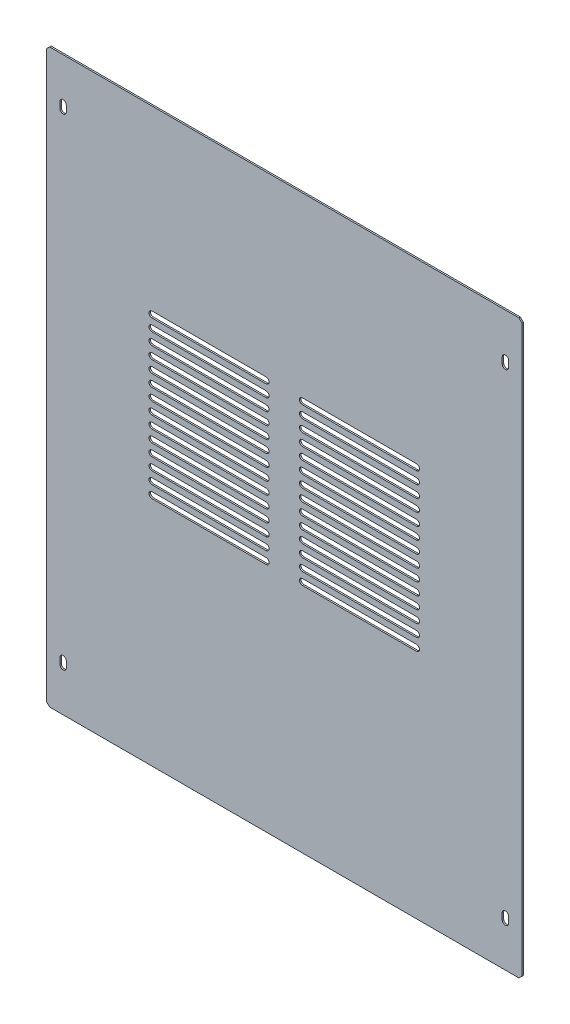
# Autodesk Inventor part: Part119
Saved by Autodesk Inventor 2016 (Build 200138000, 138)
## iProperties
Created: 2018-11-16
Part Number: Part119
Material: Generic
Document SubType Name: Sheet Metal
Designer: hovm
Density: 1 g/cm^3
Sheet Metal Rule: Default_mm
Appearance: Default
Author: hovm
Autodesk Inventor part; units mm, degrees
ref_plane "YZ Plane" through (0, 0, 0) normal (1, 0, 0) x (0, 1, 0)
ref_plane "XZ Plane" through (0, 0, 0) normal (0, 1, 0) x (-1, 0, 0)
ref_plane "XY Plane" through (0, 0, 0) normal (0, 0, 1) x (1, 0, 0)
sketch "Sketch1" plane through (0, 0, 0) normal (0, 0, 1) x (1, 0, 0)
  line L0 (-56, 475) -> (-366, 475)
  line L1 (-366, 849) -> (-56, 849)
  line L2 (-56, 889) -> (-56, 425.8173)
  line L3 (-366, 425.8173) -> (-366, 889)
  line L4 (-53, 852) -> (-369, 852)
  line L5 (-369, 852) -> (-369, 472)
  line L6 (-369, 472) -> (-53, 472)
  line L7 (-53, 472) -> (-53, 852)
  point P0 (0, 0)
  dimension "d0" = 3
  dimension "d1" = 3
  dimension "d2" = 3
  dimension "d33" = 3
  measures "d0" distance between parallel lines of L1 L4
  measures "d1" distance between parallel lines of L3 L5
  measures "d2" distance between parallel lines of L0 L6
  measures "d33" distance between parallel lines of L2 L7
extrude "Plate1" add sketch "Sketch1" along normal blind 1
chamfer "Corner Chamfer1" distance 2 angle 45 4 edges at (-53, 852, 0.5) (-369, 852, 0.5) (-369, 472, 0.5) (-53, 472, 0.5)
sketch "Sketch3" plane through (0, 0, 0) normal (0, 0, -1) x (-1, 0, 0)
  circle A0 centre (64, 822) radius 1.5 construction
  circle A1 centre (358, 502) radius 1.5 construction
  circle A2 centre (358, 822) radius 1.5 construction
  circle A3 centre (64, 502) radius 1.5 construction
  line L0 (64, 824) -> (64, 820) construction
  line L1 (61.8, 824) -> (61.8, 820)
  line L2 (66.2, 820) -> (66.2, 824)
  arc A4 (66.2, 824) -> (61.8, 824) centre (64, 824) ccw
  arc A5 (61.8, 820) -> (66.2, 820) centre (64, 820) ccw
  line L3 (358, 824) -> (358, 820) construction
  line L4 (355.8, 824) -> (355.8, 820)
  line L5 (360.2, 820) -> (360.2, 824)
  arc A6 (360.2, 824) -> (355.8, 824) centre (358, 824) ccw
  arc A7 (355.8, 820) -> (360.2, 820) centre (358, 820) ccw
  line L6 (358, 504) -> (358, 500) construction
  line L7 (355.8, 504) -> (355.8, 500)
  line L8 (360.2, 500) -> (360.2, 504)
  arc A8 (360.2, 504) -> (355.8, 504) centre (358, 504) ccw
  arc A9 (355.8, 500) -> (360.2, 500) centre (358, 500) ccw
  line L9 (64, 504) -> (64, 500) construction
  line L10 (61.8, 504) -> (61.8, 500)
  line L11 (66.2, 500) -> (66.2, 504)
  arc A10 (66.2, 504) -> (61.8, 504) centre (64, 504) ccw
  arc A11 (61.8, 500) -> (66.2, 500) centre (64, 500) ccw
  point P0 (0, 0)
  point P1 (64, 502)
  dimension "d34" = 4
  dimension "d35" = 2.2
  dimension "d36" = 4
  dimension "d37" = 2.2
  dimension "d38" = 4
  dimension "d39" = 2.2
  dimension "d40" = 4
  dimension "d41" = 2.2
  constraints: 32 end point, 16 point on circle, 16 tangent, 8 centre point, 4 midpoint, 4 parallel, 4 vertical, 3 coincident
  measures "d34" distance of L2.start L2.end
  measures "d35" radius of A4
  measures "d36" distance of L5.start L5.end
  measures "d37" radius of A6
  measures "d38" distance of L8.start L8.end
  measures "d39" radius of A8
  measures "d40" distance of L11.start L11.end
  measures "d41" radius of A10
extrude "Cut2" cut sketch "Sketch3" against normal blind 1
sketch "Sketch4" plane through (0, 0, 0) normal (0, 0, -1) x (-1, 0, 0)
  line L0 (55, 852) -> (367, 852) construction
  line L1 (211, 852) -> (211, 466.5332) construction
  line L2 (123, 732) -> (199, 732) construction
  line L3 (123, 730) -> (199, 730)
  line L4 (199, 734) -> (123, 734)
  arc A0 (123, 734) -> (123, 730) centre (123, 732) ccw
  arc A1 (199, 730) -> (199, 734) centre (199, 732) ccw
  line L5 (223, 732) -> (299, 732) construction
  line L6 (223, 730) -> (299, 730)
  line L7 (299, 734) -> (223, 734)
  arc A2 (223, 734) -> (223, 730) centre (223, 732) ccw
  arc A3 (299, 730) -> (299, 734) centre (299, 732) ccw
  line L8 (123, 724) -> (199, 724) construction
  line L9 (123, 722) -> (199, 722)
  line L10 (199, 726) -> (123, 726)
  arc A4 (123, 726) -> (123, 722) centre (123, 724) ccw
  arc A5 (199, 722) -> (199, 726) centre (199, 724) ccw
  line L11 (223, 724) -> (299, 724) construction
  line L12 (223, 722) -> (299, 722)
  line L13 (299, 726) -> (223, 726)
  arc A6 (223, 726) -> (223, 722) centre (223, 724) ccw
  arc A7 (299, 722) -> (299, 726) centre (299, 724) ccw
  line L14 (123, 716) -> (199, 716) construction
  line L15 (123, 714) -> (199, 714)
  line L16 (199, 718) -> (123, 718)
  arc A8 (123, 718) -> (123, 714) centre (123, 716) ccw
  arc A9 (199, 714) -> (199, 718) centre (199, 716) ccw
  line L17 (223, 716) -> (299, 716) construction
  line L18 (223, 714) -> (299, 714)
  line L19 (299, 718) -> (223, 718)
  arc A10 (223, 718) -> (223, 714) centre (223, 716) ccw
  arc A11 (299, 714) -> (299, 718) centre (299, 716) ccw
  line L20 (123, 708) -> (199, 708) construction
  line L21 (123, 706) -> (199, 706)
  line L22 (199, 710) -> (123, 710)
  arc A12 (123, 710) -> (123, 706) centre (123, 708) ccw
  arc A13 (199, 706) -> (199, 710) centre (199, 708) ccw
  line L23 (223, 708) -> (299, 708) construction
  line L24 (223, 706) -> (299, 706)
  line L25 (299, 710) -> (223, 710)
  arc A14 (223, 710) -> (223, 706) centre (223, 708) ccw
  arc A15 (299, 706) -> (299, 710) centre (299, 708) ccw
  line L26 (123, 700) -> (199, 700) construction
  line L27 (123, 698) -> (199, 698)
  line L28 (199, 702) -> (123, 702)
  arc A16 (123, 702) -> (123, 698) centre (123, 700) ccw
  arc A17 (199, 698) -> (199, 702) centre (199, 700) ccw
  line L29 (223, 700) -> (299, 700) construction
  line L30 (223, 698) -> (299, 698)
  line L31 (299, 702) -> (223, 702)
  arc A18 (223, 702) -> (223, 698) centre (223, 700) ccw
  arc A19 (299, 698) -> (299, 702) centre (299, 700) ccw
  line L32 (123, 692) -> (199, 692) construction
  line L33 (123, 690) -> (199, 690)
  line L34 (199, 694) -> (123, 694)
  arc A20 (123, 694) -> (123, 690) centre (123, 692) ccw
  arc A21 (199, 690) -> (199, 694) centre (199, 692) ccw
  line L35 (223, 692) -> (299, 692) construction
  line L36 (223, 690) -> (299, 690)
  line L37 (299, 694) -> (223, 694)
  arc A22 (223, 694) -> (223, 690) centre (223, 692) ccw
  arc A23 (299, 690) -> (299, 694) centre (299, 692) ccw
  line L38 (123, 684) -> (199, 684) construction
  line L39 (123, 682) -> (199, 682)
  line L40 (199, 686) -> (123, 686)
  arc A24 (123, 686) -> (123, 682) centre (123, 684) ccw
  arc A25 (199, 682) -> (199, 686) centre (199, 684) ccw
  line L41 (223, 684) -> (299, 684) construction
  line L42 (223, 682) -> (299, 682)
  line L43 (299, 686) -> (223, 686)
  arc A26 (223, 686) -> (223, 682) centre (223, 684) ccw
  arc A27 (299, 682) -> (299, 686) centre (299, 684) ccw
  line L44 (123, 676) -> (199, 676) construction
  line L45 (123, 674) -> (199, 674)
  line L46 (199, 678) -> (123, 678)
  arc A28 (123, 678) -> (123, 674) centre (123, 676) ccw
  arc A29 (199, 674) -> (199, 678) centre (199, 676) ccw
  line L47 (223, 676) -> (299, 676) construction
  line L48 (223, 674) -> (299, 674)
  line L49 (299, 678) -> (223, 678)
  arc A30 (223, 678) -> (223, 674) centre (223, 676) ccw
  arc A31 (299, 674) -> (299, 678) centre (299, 676) ccw
  line L50 (123, 668) -> (199, 668) construction
  line L51 (123, 666) -> (199, 666)
  line L52 (199, 670) -> (123, 670)
  arc A32 (123, 670) -> (123, 666) centre (123, 668) ccw
  arc A33 (199, 666) -> (199, 670) centre (199, 668) ccw
  line L53 (223, 668) -> (299, 668) construction
  line L54 (223, 666) -> (299, 666)
  line L55 (299, 670) -> (223, 670)
  arc A34 (223, 670) -> (223, 666) centre (223, 668) ccw
  arc A35 (299, 666) -> (299, 670) centre (299, 668) ccw
  line L56 (123, 660) -> (199, 660) construction
  line L57 (123, 658) -> (199, 658)
  line L58 (199, 662) -> (123, 662)
  arc A36 (123, 662) -> (123, 658) centre (123, 660) ccw
  arc A37 (199, 658) -> (199, 662) centre (199, 660) ccw
  line L59 (223, 660) -> (299, 660) construction
  line L60 (223, 658) -> (299, 658)
  line L61 (299, 662) -> (223, 662)
  arc A38 (223, 662) -> (223, 658) centre (223, 660) ccw
  arc A39 (299, 658) -> (299, 662) centre (299, 660) ccw
  line L62 (123, 652) -> (199, 652) construction
  line L63 (123, 650) -> (199, 650)
  line L64 (199, 654) -> (123, 654)
  arc A40 (123, 654) -> (123, 650) centre (123, 652) ccw
  arc A41 (199, 650) -> (199, 654) centre (199, 652) ccw
  line L65 (223, 652) -> (299, 652) construction
  line L66 (223, 650) -> (299, 650)
  line L67 (299, 654) -> (223, 654)
  arc A42 (223, 654) -> (223, 650) centre (223, 652) ccw
  arc A43 (299, 650) -> (299, 654) centre (299, 652) ccw
  line L68 (123, 644) -> (199, 644) construction
  line L69 (123, 642) -> (199, 642)
  line L70 (199, 646) -> (123, 646)
  arc A44 (123, 646) -> (123, 642) centre (123, 644) ccw
  arc A45 (199, 642) -> (199, 646) centre (199, 644) ccw
  line L71 (223, 644) -> (299, 644) construction
  line L72 (223, 642) -> (299, 642)
  line L73 (299, 646) -> (223, 646)
  arc A46 (223, 646) -> (223, 642) centre (223, 644) ccw
  arc A47 (299, 642) -> (299, 646) centre (299, 644) ccw
  line L74 (123, 636) -> (199, 636) construction
  line L75 (123, 634) -> (199, 634)
  line L76 (199, 638) -> (123, 638)
  arc A48 (123, 638) -> (123, 634) centre (123, 636) ccw
  arc A49 (199, 634) -> (199, 638) centre (199, 636) ccw
  line L77 (223, 636) -> (299, 636) construction
  line L78 (223, 634) -> (299, 634)
  line L79 (299, 638) -> (223, 638)
  arc A50 (223, 638) -> (223, 634) centre (223, 636) ccw
  arc A51 (299, 634) -> (299, 638) centre (299, 636) ccw
  line L80 (123, 628) -> (199, 628) construction
  line L81 (123, 626) -> (199, 626)
  line L82 (199, 630) -> (123, 630)
  arc A52 (123, 630) -> (123, 626) centre (123, 628) ccw
  arc A53 (199, 626) -> (199, 630) centre (199, 628) ccw
  line L83 (223, 628) -> (299, 628) construction
  line L84 (223, 626) -> (299, 626)
  line L85 (299, 630) -> (223, 630)
  arc A54 (223, 630) -> (223, 626) centre (223, 628) ccw
  arc A55 (299, 626) -> (299, 630) centre (299, 628) ccw
  point P0 (0, 0)
  point P1 (161, 732)
  point P2 (261, 732)
  point P3 (161, 724)
  point P4 (261, 724)
  point P5 (161, 716)
  point P6 (261, 716)
  point P7 (161, 708)
  point P8 (261, 708)
  point P9 (161, 700)
  point P10 (261, 700)
  point P11 (161, 692)
  point P12 (261, 692)
  point P13 (161, 684)
  point P14 (261, 684)
  point P15 (161, 676)
  point P16 (261, 676)
  point P17 (161, 668)
  point P18 (261, 668)
  point P19 (161, 660)
  point P20 (261, 660)
  point P21 (161, 652)
  point P22 (261, 652)
  point P23 (161, 644)
  point P24 (261, 644)
  point P25 (161, 636)
  point P26 (261, 636)
  point P27 (161, 628)
  point P28 (261, 628)
  dimension "d44" = 76
  dimension "d45" = 2
  dimension "d46" = 50
  dimension "d47" = 120
  dimension "d50" = 100
  dimension "d53" = 8
  constraints: 226 end point, 112 point on circle, 56 centre point, 4 tangent, 2 horizontal, 2 midpoint, 2 vertical, 1 parallel, 324 other
  measures "d44" distance of L4.start L4.end
  measures "d45" radius of A1
  measures "d46" distance from line of L1 point (161, 732)
  measures "d47" distance from line of L0 point (161, 732)
  measures "d50" distance of L3.start L6.start
  measures "d53" distance of L3.start L9.start
extrude "Cut3" cut sketch "Sketch4" against normal blind 1
equation "\"d42\" = Thickness"
equation "\"d56\" = Thickness"
equation "\"BendRadius\" = Thickness"
equation "\"BendReliefWidth\" = Thickness"
equation "\"BendReliefDepth\" = 0.5 * Thickness"
equation "\"CornerReliefSize\" = 4 * Thickness"
equation "\"MinimumRemnant\" = 2 * Thickness"
equation "\"TransitionRadius\" = BendRadius"
equation "\"JacobiRadiusSize\" = BendRadius"
equation "\"GapSize\" = Thickness"
equation "\"d4\" = BendRadius"
equation "\"Thickness\" = 1"
body "Solid1"
